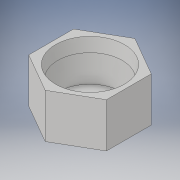
# Autodesk Inventor part: Part2
Saved by Autodesk Inventor 2019.4 (Build 234330000, 330)
## iProperties
Created: 2020-04-26
Part Number: Part2
Material: Generic
Document SubType Name: Modeling
Designer: Cedric
Density: 1 g/cm^3
Appearance: Default
Author: Cedric
Autodesk Inventor part; units mm, degrees
ref_plane "YZ Plane" through (0, 0, 0) normal (1, 0, 0) x (0, 1, 0)
ref_plane "XZ Plane" through (0, 0, 0) normal (0, 1, 0) x (-1, 0, 0)
ref_plane "XY Plane" through (0, 0, 0) normal (0, 0, 1) x (1, 0, 0)
sketch "Sketch1" plane through (0, 0, 0) normal (0, 1, 0) x (-1, 0, 0)
  line L0 (-17.5, 10.1036) -> (0, 20.2073)
  line L1 (0, 20.2073) -> (17.5, 10.1036)
  line L2 (17.5, 10.1036) -> (17.5, -10.1036)
  line L3 (17.5, -10.1036) -> (0, -20.2073)
  line L4 (0, -20.2073) -> (-17.5, -10.1036)
  line L5 (-17.5, -10.1036) -> (-17.5, 10.1036)
  point P0 (0, 0)
  point P1 (0, 0)
  dimension "d0" = 35
  constraints: 12 end point, 1 coincident, 1 vertical, 13 other
  measures "d0" distance from line of L1 L3.end
extrude "Extrusion1" add sketch "Sketch1" along normal mid plane 20
sketch "Sketch2" plane through (0, 10, 0) normal (0, 1, 0) x (1, 0, 0)
  circle A0 centre (0, 0) radius 14.5
  dimension "d3" = 29
  constraints: 1 centre point, 1 coincident
  measures "d3" diameter of A0
extrude "Extrusion2" cut sketch "Sketch2" against normal blind 18
chamfer "Chamfer1" distance 1 angle 80 1 edges at (-14.5, 10, 0) measured on face at (-8.579, 10, 14.0814)
body "Solid1"
